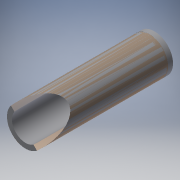
# Autodesk Inventor part: straight_fit
Saved by Autodesk Inventor 2016 (Build 200138000, 138)
## iProperties
Created: 2016-03-15
Part Number: straight_fit
Material: Generic
Document SubType Name: Modeling
Designer: GentnerLab
Density: 1 g/cm^3
Appearance: Default
Author: GentnerLab
Autodesk Inventor part; units mm, degrees
ref_plane "YZ Plane" through (0, 0, 0) normal (1, 0, 0) x (0, 1, 0)
ref_plane "XZ Plane" through (0, 0, 0) normal (0, 1, 0) x (-1, 0, 0)
ref_plane "XY Plane" through (0, 0, 0) normal (0, 0, 1) x (1, 0, 0)
sketch "Sketch1" plane through (0, 0, 0) normal (0, 0, 1) x (1, 0, 0)
  circle A0 centre (0, 0) radius 0.9525
  dimension "d0" = 1.905
  constraints: 1 centre point, 1 coincident
  measures "d0" diameter of A0
surface extrude "ExtrusionSrf1" sketch "Sketch1" along normal blind 6.35 shown yes curves A0
thicken "Thicken1" operation new thickness 0.254 both sides no extend neighbours no toward (-0.9967573, 0.0804666, 0) faces at (0.9494, -0.0766, 4.2333)
thicken "Thicken2" operation new thickness 0.254 both sides no extend neighbours no toward (0, 0, -1) faces at (0.8586, -0.076, 0)
body "Solid1"
body "Srf1"
body "Solid2"
